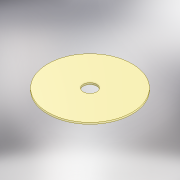
# Autodesk Inventor part: feed_lid
Saved by Autodesk Inventor 2020 (Build 240168000, 168)
## iProperties
Created: 2020-06-18
Part Number: feed_lid
Material: Generic
Document SubType Name: Modeling
Designer: pc-konvi
Density: 1 g/cm^3
Appearance: Nylon 6
Author: pc-konvi
Autodesk Inventor part; units mm, degrees
ref_plane "YZ Plane" through (0, 0, 0) normal (1, 0, 0) x (0, 1, 0)
ref_plane "XZ Plane" through (0, 0, 0) normal (0, 1, 0) x (-1, 0, 0)
ref_plane "XY Plane" through (0, 0, 0) normal (0, 0, 1) x (1, 0, 0)
sketch "Sketch1" plane through (0, 0, 0) normal (0, 0, 1) x (1, 0, 0)
  line L0 (0, 0) -> (8, 0) construction
  line L1 (8, 0) -> (8, -2) construction
  line L2 (8, -2) -> (0, -2) construction
  line L3 (0, -2) -> (0, 0) construction
  line L4 (0, 0) -> (50, 0) construction
  line L5 (8, 0) -> (50, 0)
  line L6 (50, 0) -> (50, -2)
  line L7 (50, -2) -> (8, -2)
  line L8 (8, -2) -> (8, 0)
  line L9 (44, -2) -> (46, -2)
  line L10 (46, -2) -> (46, -4)
  line L11 (46, -4) -> (44, -4)
  line L12 (44, -4) -> (44, -2)
  dimension "d0" = 8
  dimension "d1" = 2
  dimension "d2" = 50
  dimension "d3" = 2
  dimension "d4" = 2
  dimension "d5" = 4
  dimension "d6" = 42
  constraints: 26 end point, 6 parallel, 4 horizontal, 3 perpendicular, 1 point on line
  measures "d0" distance of L1.end L2.end
  measures "d1" distance of L0.end L1.end
  measures "d2" distance of L0.start L4.end
  measures "d3" distance of L10.end L11.end
  measures "d4" distance of L9.end L10.end
  measures "d5" distance between parallel lines of L6 L10
  measures "d6" distance between parallel lines of L1 L6
revolve "Revolution1" add sketch "Sketch1" angle 360 about axis through (0, -2, 0) along (0, 1, 0)
equation "\"d6\" = d2 - d0"
body "Solid1"
